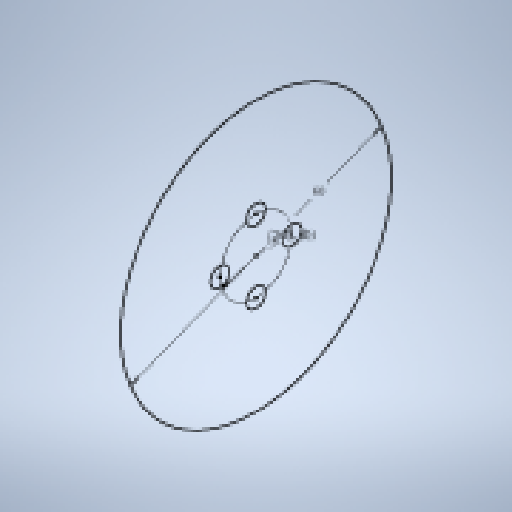
# Autodesk Inventor part: 主动轮
Saved by Autodesk Inventor 2025.1 (Build 291241000, 241)
## iProperties
Created: 2025-08-27
Part Number: 主动轮
Material: 常规
Document SubType Name: Modeling
Designer: Piw
Density: 1 g/cm^3
Appearance: 默认
Author: Piw
Autodesk Inventor part; units mm, degrees
ref_plane "YZ Plane" through (0, 0, 0) normal (1, 0, 0) x (0, 1, 0)
ref_plane "XZ Plane" through (0, 0, 0) normal (0, 1, 0) x (-1, 0, 0)
ref_plane "XY Plane" through (0, 0, 0) normal (0, 0, 1) x (1, 0, 0)
sketch "草图3" plane through (0, 0, 0) normal (1, 0, 0) x (0, 1, 0)
  circle A0 centre (0, 0) radius 8 construction
  circle A1 centre (0, -8) radius 2.1
  line L0 (0, 0) -> (0, -8) construction
  circle A2 centre (8, 0) radius 2.1
  circle A3 centre (0, 8) radius 2.1
  circle A4 centre (-8, 0) radius 2.1
  circle A5 centre (0, 0) radius 42.5
  dimension "d21" = 16
  dimension "d22" = 4.2
  dimension "d25" = 360
  dimension "d27" = 85
  constraints: 5 centre point, 2 coincident, 2 end point, 1 vertical, 1 vertical alignment, 11 other
  measures "d22" diameter of A1
  measures "d27" diameter of A5
extrude "拉伸3" add sketch "草图3" against normal blind 18.5
sketch "草图6" plane through (-18.5, 0, 0) normal (-1, 0, 0) x (0, 0, 1)
  circle A0 centre (0, 0) radius 30
  circle A1 centre (0, 0) radius 42.5 projected
  dimension "d30" = 60
  constraints: 1 centre point, 1 coincident
  measures "d30" diameter of A0
extrude "拉伸4" add sketch "草图6" along normal blind 11.5
chamfer "倒角1" distance 5 angle 45 1 edges at (-18.5, 0, -30)
sketch "草图7" plane through (0, 0, 0) normal (1, 0, 0) x (0, 0, -1)
  circle A0 centre (0, 0) radius 27.5
  circle A1 centre (0, 0) radius 42.5 projected
  dimension "d36" = 55
  constraints: 1 centre point, 1 coincident
  measures "d36" diameter of A0
extrude "拉伸5" cut sketch "草图7" against normal blind 19
chamfer "倒角2" distance 2 angle 45 1 edges at (-19, 0, 27.5)
sketch "草图8" plane through (0, 0, 0) normal (1, 0, 0) x (0, 0, -1)
  circle A0 centre (0, 0) radius 20 construction
  circle A1 centre (20, 0) radius 2.1
  line L0 (20, 0) -> (0, 0) construction
  line L1 (14.1421, 14.1421) -> (0, 0) construction
  circle A2 centre (14.1421, 14.1421) radius 2.1
  line L2 (0, 20) -> (0, 0) construction
  circle A3 centre (0, 20) radius 2.1
  line L3 (-14.1421, 14.1421) -> (0, 0) construction
  circle A4 centre (-14.1421, 14.1421) radius 2.1
  line L4 (-20, 0) -> (0, 0) construction
  circle A5 centre (-20, 0) radius 2.1
  line L5 (-14.1421, -14.1421) -> (0, 0) construction
  circle A6 centre (-14.1421, -14.1421) radius 2.1
  line L6 (0, -20) -> (0, 0) construction
  circle A7 centre (0, -20) radius 2.1
  line L7 (14.1421, -14.1421) -> (0, 0) construction
  circle A8 centre (14.1421, -14.1421) radius 2.1
  dimension "d42" = 40
  dimension "d43" = 4.2
  dimension "d46" = 360
  constraints: 16 end point, 8 centre point, 1 coincident, 1 horizontal, 1 horizontal alignment, 35 other
  measures "d43" diameter of A1
extrude "拉伸6" cut sketch "草图8" against normal through all
chamfer "倒角4" distance 1 angle 45 2 edges at (-19, 0, -42.5) (-30, 0, -42.5)
